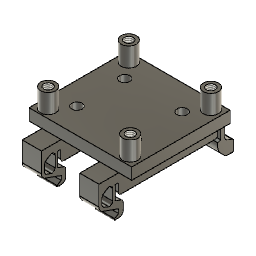
JRCNC0002 v2 (Autodesk Fusion 360 design; units mm, degrees)
Autodesk Fusion 360 part; units mm, degrees
sketch "Sketch1" plane through (0, 0, 0) normal (0, 0, 1) x (1, 0, 0)
  line L0 (13.5, 13.25) -> (-13.5, 13.25)
  line L1 (-13.5, 13.25) -> (-13.5, -13.25)
  line L2 (-13.5, -13.25) -> (13.5, -13.25)
  line L3 (13.5, -13.25) -> (13.5, 13.25)
  line L4 (13.5, 13.25) -> (-13.5, -13.25) construction
  line L5 (-13.5, 13.25) -> (13.5, -13.25) construction
  line L6 (17, 16.2766) -> (-17, 16.2766)
  line L7 (-17, 16.2766) -> (-17, -16.2766)
  line L8 (-17, -16.2766) -> (17, -16.2766)
  line L9 (17, -16.2766) -> (17, 16.2766)
  line L10 (-13.5, 13.25) -> (13.5, -13.25) construction
  line L11 (-13.5, -13.25) -> (13.5, 13.25) construction
  dimension "d4" = 26.5
  dimension "d48" = 34
  dimension "d49" = 27
  constraint horizontal L0
  constraint perpendicular L0 L1
  constraint parallel L0 L2
  constraint parallel L1 L3
  constraint coincident L4 origin
  constraint coincident L5 origin
  constraint horizontal L6
  constraint perpendicular L6 L7
  constraint parallel L6 L8
  constraint parallel L7 L9
  constraint parallel L5 L10
  measures "d4" distance of L0.end L1.end
  measures "d48" distance of L6.start L6.end
  measures "d49" distance of L0.start L0.end
extrude "Extrude1" add sketch "Sketch1" along normal blind 3.81 contours L0 L1 L2 L3 | L6 L7 L8 L9 makes body 1
sketch "Sketch4" plane through (0, 0, 3.81) normal (0, 0, 1) x (-1, 0, 0)
  line L0 (13.6, -13.35) -> (-13.6, -13.35)
  line L1 (-13.6, -13.35) -> (-13.6, 13.35)
  line L2 (-13.6, 13.35) -> (13.6, 13.35)
  line L3 (13.6, 13.35) -> (13.6, -13.35)
  line L4 (13.6, -13.35) -> (-13.6, 13.35) construction
  line L5 (-13.6, -13.35) -> (13.6, 13.35) construction
  circle A0 centre (13.6, -13.35) radius 2.5
  circle A1 centre (-13.6, -13.35) radius 2.5
  circle A2 centre (-13.6, 13.35) radius 2.5
  circle A3 centre (13.6, 13.35) radius 2.5
  line L6 (-17, -16.2766) -> (17, -16.2766)
  line L7 (17, -16.2766) -> (17, 16.2766)
  line L8 (17, 16.2766) -> (-17, 16.2766)
  line L9 (-17, 16.2766) -> (-17, -16.2766)
  dimension "d17" = 27.2
  dimension "d18" = 26.7
  dimension "d19" = 5
  constraint horizontal L0
  constraint perpendicular L0 L1
  constraint parallel L0 L2
  constraint parallel L1 L3
  constraint coincident L4 origin
  constraint coincident L5 origin
  constraint coincident L0.start L3.end
  constraint coincident L0.end L1.start
  constraint coincident L1.end L2.start
  constraint coincident L2.end L3.start
  constraint equal A2 A3
  constraint equal A1 A2
  constraint equal A0 A1
  measures "d17" distance of L0.start L0.end
  measures "d18" distance of L0.start L2.end
  measures "d19" diameter of A0
extrude "Extrude3" add sketch "Sketch4" along normal blind 6.35 contours L0 L1 A1 | L0 L1 A1 | L0 L3 A0 | L0 L3 A0 | L1 L2 A2 | L1 L2 A2 | L2 L3 A3 | L2 L3 A3 bodies 1
sketch "Sketch5" plane through (0, 0, 10.16) normal (0, 0, 1) x (-1, 0, 0)
  circle A0 centre (-13.6, -13.35) radius 2.5
  line L0 (-13.6, 13.35) -> (13.6, 13.35)
  line L1 (-13.6, -13.35) -> (-13.6, 13.35)
  line L2 (13.6, 13.35) -> (13.6, -13.35)
  line L3 (13.6, -13.35) -> (-13.6, -13.35)
hole "Hole1" at (13.6, -13.35, 10.16) at (-13.6, -13.35, 10.16) at (-13.6, 13.35, 10.16) at (13.6, 13.35, 10.16) direction (0, 0, -1) diameter 2.921 depth 50.8 tip angle 180 bodies 1
thread "Thread1" "ANSI Metric M Profile 3.5 M3.5x0.6 6H"
sketch "Sketch8" plane through (0, 0, 0) normal (1, 0, 0) x (0, 1, 0)
  line L0 (21.4875, -9.2063) -> (21.2899, -9.1344)
  arc A0 (-18.2855, -3.4183) -> (-19.7022, -2.5095) centre (-19.2852, -3.4181) ccw
  arc A1 (-14.7835, -9.1363) -> (-15.4415, -8.1964) centre (-15.7839, -9.1364) ccw
  arc A2 (-16.2835, -12.9263) -> (-14.7835, -11.4263) centre (-16.2835, -11.4263) ccw
  line L1 (17.5415, -1.9263) -> (17.5415, -7.4793)
  line L2 (-15.4585, -6.4763) -> (15.539, -6.3877)
  arc A3 (-22.8335, -6.5423) -> (-21.5176, -8.4215) centre (-20.8341, -6.5424) ccw
  arc A4 (16.4903, -7.7613) -> (17.5877, -11.3545) centre (20.4167, -8.5263) ccw
  arc A5 (21.2899, -9.1344) -> (21.2754, -9.1293) centre (21.0165, -9.8863) ccw
  line L3 (-14.7835, -11.4263) -> (-14.7835, -9.1363)
  line L4 (-16.2835, -10.3263) -> (-16.2835, -11.6763)
  line L5 (-21.8355, -6.5383) -> (-21.8355, -4.4463)
  arc A6 (-21.5105, -3.7085) -> (-21.8355, -4.4463) centre (-20.8358, -4.4462) ccw
  arc A7 (-21.8355, -6.5383) -> (-21.1776, -7.4781) centre (-20.8352, -6.5381) ccw
  arc A8 (21.3165, -12.9263) -> (21.8165, -12.4263) centre (21.3165, -12.4263) ccw
  line L6 (19.5735, -12.9263) -> (21.3165, -12.9263)
  line L7 (-16.4585, -2.9263) -> (-16.4585, -5.4763)
  line L8 (-17.4585, -7.4626) -> (-17.4585, -2.9263)
  line L9 (16.5415, -5.4763) -> (16.5415, -1.9263)
  arc A9 (21.7933, -9.5259) -> (21.4875, -9.2063) centre (21.3163, -9.6763) ccw
  line L10 (21.8165, -12.4263) -> (21.8165, -9.6763)
  arc A10 (-16.4585, -2.9263) -> (-17.4585, -2.9263) centre (-16.9585, -3.2579) ccw
  line L11 (-16.2835, -11.6763) -> (-17.6624, -12.4724)
  arc A11 (-19.7022, -2.5095) -> (-21.5105, -3.7085) centre (-16.7774, -8.8841) ccw
  line L12 (-21.5176, -8.4215) -> (-16.2835, -10.3263)
  line L13 (17.5415, -7.4793) -> (16.4903, -7.7613)
  line L14 (-15.4415, -8.1964) -> (-17.4585, -7.4626)
  line L15 (-19.6276, -8.0421) -> (-21.1776, -7.4781)
  arc A12 (18.8816, -7.5417) -> (19.5394, -8.4981) centre (19.8818, -7.5582) ccw
  arc A13 (-17.6624, -12.4724) -> (-17.5405, -12.9265) centre (-17.5406, -12.6831) ccw
  arc A14 (21.8165, -9.6763) -> (21.7933, -9.5259) centre (21.3165, -9.6763) ccw
  line L16 (-17.5405, -12.9265) -> (-16.2835, -12.9263)
  line L17 (21.2754, -9.1293) -> (19.5394, -8.4981)
  arc A15 (-16.4585, -5.4763) -> (-15.4585, -6.4763) centre (-15.4585, -5.4763) ccw
  arc A16 (-19.6276, -8.0421) -> (-18.2855, -7.1023) centre (-19.2857, -7.1022) ccw
  arc A17 (17.5415, -1.9263) -> (16.5415, -1.9263) centre (17.0415, -2.2579) ccw
  line L18 (-18.2855, -3.4183) -> (-18.2855, -7.1023)
  arc A18 (18.8664, -12.6333) -> (19.5735, -12.9263) centre (19.5734, -11.9268) ccw
  arc A19 (15.539, -6.3877) -> (16.5415, -5.4763) centre (15.5674, -5.4119) ccw
  line L19 (17.5877, -11.3545) -> (18.8664, -12.6333)
  line L20 (-29.8693, 0) -> (29.8693, 0)
  line L21 (-22.8335, -6.5423) -> (-22.833, 0)
  line L22 (18.8816, 0) -> (18.8816, -7.5417)
  line L23 (0, 0) -> (0, -0.292)
  line L24 (0, -0.292) -> (0, -15.7941)
  point P0 (0.0402, -6.432)
  constraint coincident L20 L21.end
  constraint tangent A3 L21
  constraint coincident L20 L22.start
  constraint perpendicular L20 L22
  constraint coincident L23.start origin
  constraint perpendicular L20 L23
  constraint midpoint L2 P0
extrude "Extrude7" add sketch "Sketch8" along normal blind 12.7 and the other way blind 12.7 separate body makes body 2
extrude "Extrude8" cut sketch "Sketch8" along normal mid plane 12.7 bodies 2 makes body 3 at (6.35, 5.5406, -4.9301)
sketch "Sketch9" plane through (0, 0.0184, -6.432) normal (0, 0.002857, -0.999996) x (-1, 0, 0)
  line L0 (-9.525, 7.9134) -> (9.525, 7.9134)
  line L1 (9.525, 7.9134) -> (9.525, -7.9134)
  line L2 (9.525, -7.9134) -> (-9.525, -7.9134)
  line L3 (-9.525, -7.9134) -> (-9.525, 7.9134)
  line L4 (-9.525, 7.9134) -> (9.525, -7.9134) construction
  line L5 (9.525, 7.9134) -> (-9.525, -7.9134) construction
  line L6 (-6.35, 7.9134) -> (-12.7, 7.9134)
  line L7 (-12.7, -15.477) -> (-12.7, 15.5207)
  line L8 (-6.35, -15.477) -> (-6.35, 15.5207)
  constraint horizontal L0
  constraint perpendicular L0 L1
  constraint parallel L0 L2
  constraint parallel L1 L3
  constraint coincident L4 origin
  constraint coincident L5 origin
  constraint parallel L0 L6
  constraint coincident L6.end L7
  constraint coincident L6.start L8
  constraint midpoint L0.start L6
hole "Hole2" at (9.525, 7.9317, -6.4094) at (9.525, -7.895, -6.4546) at (-9.525, 7.9317, -6.4094) at (-9.525, -7.895, -6.4546) direction (0, -0.002857, 0.999996) diameter 2.921 depth 50.8 tip angle 180 bodies 1 2 3
thread "Thread2" "ANSI Metric M Profile 3.5 M3.5x0.6 6H"
sketch "Sketch10" plane through (0, 0, 3.81) normal (0, 0, 1) x (-1, 0, 0)
  ellipse E0 centre (9.525, -7.9025) end of major axis (9.525, -6.4375) minor radius 1.465
  ellipse E1 centre (-9.525, -7.9025) end of major axis (-9.525, -6.4375) minor radius 1.465
  ellipse E2 centre (-9.525, 7.9243) end of major axis (-9.525, 9.3893) minor radius 1.465
  ellipse E3 centre (9.525, 7.9243) end of major axis (9.525, 9.3893) minor radius 1.465
  circle A0 centre (-13.6, -13.35) radius 2.5
  circle A1 centre (-13.6, 13.35) radius 2.5
  circle A2 centre (13.6, -13.35) radius 2.5
  circle A3 centre (13.6, 13.35) radius 2.5
  line L0 (-17, 16.2766) -> (-17, -16.2766)
  line L1 (-17, -16.2766) -> (17, -16.2766)
  line L2 (17, -16.2766) -> (17, 16.2766)
  line L3 (17, 16.2766) -> (-17, 16.2766)
  line L4 (9.525, 7.895) -> (-9.525, 7.895)
  line L5 (9.525, -7.9317) -> (9.525, 7.895)
  line L6 (-9.525, -7.9317) -> (9.525, -7.9317)
  line L7 (-9.525, 7.895) -> (-9.525, -7.9317)
hole "Hole4" at (9.525, 7.9317, 3.81) at (-9.525, 7.9317, 3.81) at (9.525, -7.895, 3.81) at (-9.525, -7.895, 3.81) direction (0, 0, -1) diameter 3.4036 end up to surface (3.81 mm away) bodies 1
